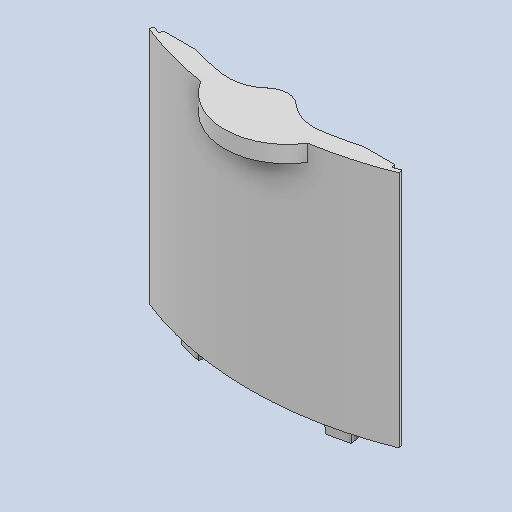
# Autodesk Inventor part: battery_lid
Saved by Autodesk Inventor 2025 (Build 290162000, 162)
## iProperties
Created: 2026-03-20
Part Number: battery_lid
Material: Generic
Document SubType Name: Modeling
Designer: Luca
Density: 1 g/cm^3
Appearance: Default
Author: Luca
Autodesk Inventor part; units mm, degrees
ref_plane "YZ Plane" through (0, 0, 0) normal (1, 0, 0) x (0, 1, 0)
ref_plane "XZ Plane" through (0, 0, 0) normal (0, 1, 0) x (-1, 0, 0)
ref_plane "XY Plane" through (0, 0, 0) normal (0, 0, 1) x (1, 0, 0)
derived "sk_reservoir.ipt"
sketch "battery_lid" plane through (0, -57.9, 0) normal (0, 1, 0) x (-1, 0, 0)
  arc A0 (38.25, -67.9775) -> (-67.9775, 38.25) centre (0, 0) ccw construction
  line L0 (0, -80) -> (0, 80) construction
  circle A1 centre (0, 0) radius 80
  arc A2 (-14.9031, 77.5816) -> (-20.7481, 76.2267) centre (0, 0) ccw
  arc A3 (-14.2257, 74.659) -> (-20.0707, 73.3042) centre (0, 0) ccw
  line L1 (-17.1615, 74.0393) -> (-17.8385, 76.9597) construction
  line L2 (-14.9031, 77.5816) -> (-14.2257, 74.659)
  line L3 (-20.0707, 73.3042) -> (-20.7481, 76.2267)
  arc A4 (20.2646, 72.9914) -> (-20.2646, 72.9914) centre (0, 0) ccw
  line L4 (20.2646, 72.9914) -> (21.4009, 77.0844)
  line L5 (-20.2646, 72.9914) -> (-21.4009, 77.0844)
  line L6 (-14.5278, 74.8555) -> (-15.0922, 77.2903)
  line L7 (-19.8858, 73.6136) -> (-20.4501, 76.0484)
  arc A5 (-14.5278, 74.8555) -> (-19.8858, 73.6136) centre (0, 0) ccw
  arc A6 (-15.0922, 77.2903) -> (-20.4501, 76.0484) centre (0, 0) ccw
  line L8 (25, 80) -> (-25, 80) construction
  line L9 (14.5278, 74.8555) -> (15.0922, 77.2903)
  arc A7 (20.4501, 76.0484) -> (15.0922, 77.2903) centre (0, 0) ccw
  line L10 (19.8858, 73.6136) -> (20.4501, 76.0484)
  arc A8 (19.8858, 73.6136) -> (14.5278, 74.8555) centre (0, 0) ccw
  arc A9 (20.7481, 76.2267) -> (14.9031, 77.5816) centre (0, 0) ccw
  line L11 (17.1615, 74.0393) -> (17.8385, 76.9597) construction
  arc A10 (20.0707, 73.3042) -> (14.2257, 74.659) centre (0, 0) ccw
  line L12 (20.0707, 73.3042) -> (20.7481, 76.2267)
  line L13 (14.9031, 77.5816) -> (14.2257, 74.659)
  line L14 (-27.5, 72.9914) -> (-20.2646, 72.9914)
  line L15 (20.2646, 72.9914) -> (27.5, 72.9914)
  arc A11 (-4.983, 75.5882) -> (4.983, 75.5882) centre (0, 76) ccw
  circle A12 centre (0, 76) radius 3
  arc A13 (12.7529, 78.977) -> (-12.7529, 78.977) centre (0, 71.0799) ccw
  line L16 (-29.5024, 73.2792) -> (-29.8776, 74.2114)
  line L17 (29.5024, 73.2792) -> (29.8776, 74.2114)
  line L18 (27.879, 73.9328) -> (27.5, 72.9914)
  line L19 (-27.879, 73.9328) -> (-27.5, 72.9914)
  line L20 (-28.0175, 73.6075) -> (-27.6688, 72.7414)
  line L21 (28.0175, 73.6075) -> (27.6688, 72.7414)
  line L22 (29.6409, 72.9539) -> (30.1094, 74.1176)
  line L23 (-29.6409, 72.9539) -> (-30.1094, 74.1176)
  line L24 (-20.0936, 71.7414) -> (-28.3442, 71.7414)
  line L25 (28.3442, 71.7414) -> (20.0936, 71.7414)
  arc A14 (-5.2026, 75.296) -> (5.2026, 75.296) centre (0, 76) ccw
  line L26 (31.0336, 73.7355) -> (30.1951, 71.6528)
  line L27 (30.1951, 71.6528) -> (28.5717, 72.3064)
  line L28 (-31.0336, 73.7355) -> (-30.1951, 71.6528)
  line L29 (-30.1951, 71.6528) -> (-28.5717, 72.3064)
  line L30 (-28.5717, 72.3064) -> (-28.3442, 71.7414)
  line L31 (28.5717, 72.3064) -> (28.3442, 71.7414)
  line L32 (-29.5024, 73.2792) -> (-27.879, 73.9328)
  line L33 (-29.6409, 72.9539) -> (-28.0175, 73.6075)
  line L34 (-29.0642, 74.5337) -> (-28.3172, 72.6783) construction
  line L35 (29.0642, 74.5337) -> (28.3172, 72.6783) construction
  line L36 (28.0175, 73.6075) -> (29.6409, 72.9539)
  line L37 (29.5024, 73.2792) -> (27.879, 73.9328)
  arc A15 (20.2305, 72.7414) -> (-20.2305, 72.7414) centre (0, 0) ccw
  line L38 (27.6688, 72.7414) -> (20.2305, 72.7414)
  line L39 (-27.6688, 72.7414) -> (-20.2305, 72.7414)
  line L40 (28.5717, 72.3064) -> (27.4912, 72.7414)
  line L41 (-28.5717, 72.3064) -> (-27.4912, 72.7414)
  arc A16 (20.0936, 71.7414) -> (-20.0936, 71.7414) centre (0, 0) ccw
  line L42 (28.5717, 72.3064) -> (28.9452, 73.234)
  line L43 (-28.5717, 72.3064) -> (-28.9452, 73.234)
  point P0 (-68.9797, 38.25)
  point P1 (-25, 80)
  point P2 (25, 80)
  point P3 (-17.5, 75.4995)
  point P4 (17.5, 75.4995)
  point P5 (17.5, 75.4995)
  point P6 (-24.5, 52.3355)
  point P7 (24.5, 52.3355)
  point P8 (4.6418, 56.0699)
  point P9 (-4.6418, 56.0699)
  point P10 (-12.7529, 78.977)
  point P11 (12.7529, 78.977)
  point P12 (4.983, 75.5882)
  point P13 (-4.983, 75.5882)
  point P14 (-29.8776, 74.2114)
  point P15 (29.8776, 74.2114)
  point P16 (-28.6907, 73.606)
  point P17 (28.6907, 73.606)
  point P18 (0, 0)
  point P19 (2.9843, 75.6934)
  point P20 (-2.9843, 75.6934)
  point P21 (4.9562, 75.3394)
  point P22 (2.9482, 75.4447)
ref_plane "hull_mount_top" through (0, -57.9, 0) normal (0, 1, 0) x (-1, 0, 0)
ref_plane "battery_lid_top" through (0, -1, 0) normal (0, 1, 0) x (-1, 0, 0)
ref_plane "Work Plane26" through (0, -3, 0) normal (0, 1, 0) x (-1, 0, 0)
extrude "Extrusion1" add sketch "battery_lid" along normal up to surface (56.9 mm away) from surface at 0 contours L17 L37 L18 L15 L4 A1 | A1 L5 L14 L19 L32 L16 | L4 A4 A12 L5 A1 | A4 A12 | L2 A3 L3 A2 | A5 L7 A6 L6 | L9 A7 L10 A8 | L12 A10 L13 A9
extrude "Extrusion2" add sketch "battery_lid" against normal blind 3 contours A5 L7 A6 L6 | L9 A7 L10 A8
chamfer "Chamfer1" distance 0.15 distance2 3 4 edges at (17.782, -60.9, 76.7161) (14.81, -60.9, 76.0729) (20.168, -60.9, 74.831) (17.218, -60.9, 74.2829) measured on face at (15.2971, -60.9, 75.96) measured on face at (17.6691, -60.9, 76.229) measured on face at (19.6809, -60.9, 74.9439) measured on face at (17.3309, -60.9, 74.77)
chamfer "Chamfer2" distance 0.15 distance2 3 4 edges at (-17.782, -60.9, 76.7161) (-14.81, -60.9, 76.0729) (-17.218, -60.9, 74.2829) (-20.168, -60.9, 74.831) measured on face at (-15.2971, -60.9, 75.96) measured on face at (-17.3309, -60.9, 74.77) measured on face at (-17.6691, -60.9, 76.229) measured on face at (-19.6809, -60.9, 74.9439)
extrude "Extrusion4" add sketch "battery_lid" against normal blind 4 from surface at 56.9 contours A11 A15 A12 A4 | A11 A16 A12 A15 | A4 A12 A15 A11 | A15 A12 A16 A11 | A12 A15 A4 | A11 A16 A12 | A12 A16 A15 | A12 A16
extrude "Extrusion5" cut sketch "battery_lid" along normal mid plane 2.5 from surface at 54.9 contours A12 A15 A4 | A4 A12 | A12 A16 A15 | A12 A16
extrude "Extrusion6" add sketch "battery_lid" against normal blind 4 from surface at 56.9 contours A1 A13
fillet "Fillet1" radius 10 2 edges at (-4.983, -3, 75.5882) (4.983, -3, 75.5882)
body "Solid1"
